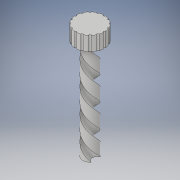
# Autodesk Inventor part: Part1
Saved by Autodesk Inventor 2019 (Build 230136000, 136)
## iProperties
Created: 2021-01-20
Part Number: Part1
Material: Generic
Document SubType Name: Modeling
Designer: kimsl
Density: 1 g/cm^3
Appearance: Default
Author: kimsl
Autodesk Inventor part; units mm, degrees
ref_plane "YZ Plane" through (0, 0, 0) normal (1, 0, 0) x (0, 1, 0)
ref_plane "XZ Plane" through (0, 0, 0) normal (0, 1, 0) x (-1, 0, 0)
ref_plane "XY Plane" through (0, 0, 0) normal (0, 0, 1) x (1, 0, 0)
sketch "Sketch1" plane through (0, 0, 0) normal (0, 1, 0) x (-1, 0, 0)
  circle A0 centre (0, 0) radius 7.5
  dimension "d0" = 15
  constraints: 1 centre point, 1 coincident
  measures "d0" diameter of A0
extrude "Extrusion1" add sketch "Sketch1" along normal blind 120
sketch "Sketch3" plane through (0, 0, 0) normal (0, -1, 0) x (1, 0, 0)
  circle A0 centre (0, 0) radius 7.5 projected
  circle A1 centre (-7.5, 0) radius 5
  dimension "d12" = 10
  constraints: 2 horizontal alignment, 1 centre point, 1 other
  measures "d12" diameter of A1
sketch "Sketch3 outline for Coil2" plane through (0, 0, 0) normal (0, -1, 0) x (1, 0, 0)
  circle A0 centre (-7.5, 0) radius 5
coil "Coil2" sketch "Sketch3 outline for Coil2" operation cut axis through (0, -10, 0) along (0, 1, 0) pitch 50 turns 2 hand left
pattern_circular "Circular Pattern1" count 2 over 360 about axis through (0, -10, 0) along (0, 1, 0) of "Coil2"
sketch "Sketch4" plane through (0, 120, 0) normal (0, 1, 0) x (1, 0, 0)
  circle A0 centre (0, 0) radius 15
  dimension "d24" = 30
  constraints: 1 centre point, 1 coincident
  measures "d24" diameter of A0
extrude "Extrusion2" add sketch "Sketch4" against normal blind 15
sketch "Sketch5" plane through (0, 120, 0) normal (0, 1, 0) x (1, 0, 0)
  circle A0 centre (0, 0) radius 15 projected
  circle A1 centre (15, 0) radius 1
  dimension "d27" = 2
  constraints: 2 horizontal alignment, 1 centre point, 1 other
  measures "d27" diameter of A1
extrude "Extrusion3" cut sketch "Sketch5" against normal blind 15 contours A0 A1 | A0 A1 picked at (14.686193, -0.226923) picked at (15.297697, -0.258605)
pattern_circular "Circular Pattern2" count 16 over 360 about axis through (0, -10, 0) along (0, 1, 0) of "Extrusion3"
body "Solid1"
